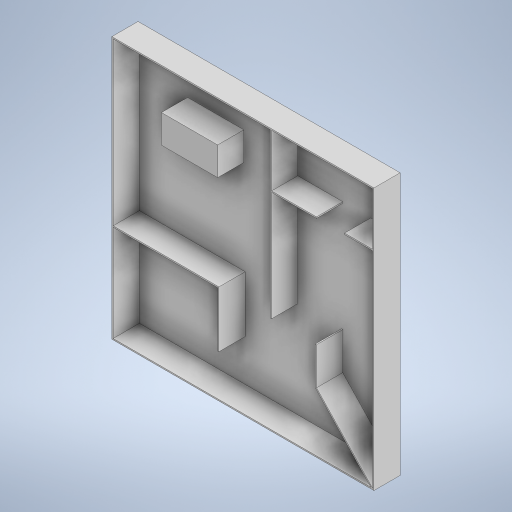
# Autodesk Inventor part: stanza_nuova_quadrata
Saved by Autodesk Inventor 2024 (Build 280153000, 153)
## iProperties
Created: 2024-04-26
Part Number: stanza_nuova_quadrata
Material: Generico
Document SubType Name: Modeling
Designer: matte
Density: 1 g/cm^3
Appearance: Default
Author: matte
Autodesk Inventor part; units mm, degrees
ref_plane "YZ Plane" through (0, 0, 0) normal (1, 0, 0) x (0, 1, 0)
ref_plane "XZ Plane" through (0, 0, 0) normal (0, 1, 0) x (-1, 0, 0)
ref_plane "XY Plane" through (0, 0, 0) normal (0, 0, 1) x (1, 0, 0)
sketch "Schizzo1" plane through (0, 0, 0) normal (0, 0, 1) x (1, 0, 0)
  line L0 (0, 0) -> (10000, 0)
  line L1 (0, 0) -> (-10000, 0)
  line L2 (-10000, 0) -> (-10000, 20000)
  line L3 (-10000, 20000) -> (10000, 20000)
  line L4 (10000, 20000) -> (10000, 0)
  line L5 (9900, 19900) -> (-9900, 19900)
  line L6 (-9900, 19900) -> (-9900, 100)
  line L7 (-9900, 100) -> (0, 100)
  line L8 (0, 100) -> (9900, 100)
  line L9 (9900, 100) -> (9900, 19900)
  line L10 (-1925, 7447) -> (-9900, 7447)
  line L11 (2190, 7447) -> (2190, 19900)
  line L12 (-1925, 7447) -> (-1925, 3264)
  line L13 (-6212, 14717) -> (-1925, 14717)
  line L14 (-1925, 14717) -> (-1925, 16877)
  line L15 (-1925, 16877) -> (-6212, 16877)
  line L16 (-6212, 16877) -> (-6212, 14717)
  line L17 (9900, 100) -> (5619, 4601)
  line L18 (5619, 4601) -> (5619, 7447)
  line L19 (2190, 15797) -> (5619, 15797)
  line L20 (7759.5, 15797) -> (9900, 15797)
  line L21 (-9900, 7547) -> (-1825, 7547)
  line L22 (-1825, 7547) -> (-1825, 3264)
  line L23 (9827.5407, 31.0823) -> (5519, 4561.0383)
  line L24 (5519, 4561.0383) -> (5519, 7447)
  line L25 (2090, 7447) -> (2090, 19900)
  line L26 (2190, 15897) -> (5619, 15897)
  line L27 (7759.5, 15897) -> (9900, 15897)
  line L28 (-1925, 3264) -> (-1825, 3264)
  line L29 (2090, 7447) -> (2190, 7447)
  line L30 (5519, 7447) -> (5619, 7447)
  line L31 (5619, 15897) -> (5619, 15797)
  line L32 (7759.5, 15897) -> (7759.5, 15797)
  point P0 (9761.9916, 100)
  dimension "d0" = 10000
  dimension "d1" = 10000
  dimension "d2" = 20000
  dimension "d3" = 20000
  dimension "d4" = 100
  dimension "d5" = 100
  dimension "d6" = 100
  dimension "d7" = 100
  dimension "d8" = 100
  dimension "d9" = 100
  constraints: 66 end point, 8 perpendicular, 7 parallel, 6 horizontal, 5 point on line, 2 vertical, 6 other
  measures "d0" distance of L0.start L0.end
  measures "d1" distance of L0.start L1.end
  measures "d2" distance of L1.end L2.end
  measures "d3" distance of L2.end L3.end
  measures "d4" distance between parallel lines of L3 L5
  measures "d5" distance between parallel lines of L10 L21
  measures "d6" distance between parallel lines of L17 L23
  measures "d7" distance between parallel lines of L11 L25
  measures "d8" distance between parallel lines of L19 L26
  measures "d9" distance between parallel lines of L20 L27
extrude "Estrusione1" add sketch "Schizzo1" along normal blind 2000 contours L1 L2 L3 L4 L0 | L11 L29 L25 L5 | L9 L20 L32 L27 | L26 L31 L19 L11 | L8 L23 L24 L30 L18 L17 | L21 L22 L28 L12 L10 L6 | L16 L15 L14 L13
sketch "Schizzo2" plane through (0, 0, 0) normal (0, 0, -1) x (-1, 0, 0)
  line L0 (-10000, 0) -> (-10000, 20000) projected
  line L1 (10000, 0) -> (-10000, 0) projected
  line L2 (-10000, 20000) -> (10000, 20000)
  line L3 (10000, 20000) -> (10000, 0)
  line L4 (10000, 0) -> (-10000, 0)
  line L5 (-10000, 0) -> (-10000, 20000)
  point P0 (0, 0)
  constraints: 8 end point, 2 parallel, 1 horizontal, 1 perpendicular
extrude "Estrusione2" add sketch "Schizzo2" against normal blind 1
